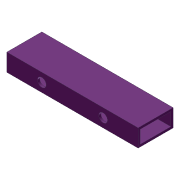
# Autodesk Inventor part: SpatulaPivotMount
Saved by Autodesk Inventor 2012 (Build 160160000, 160)
## iProperties
Created: 2013-01-18
Part Number: SpatulaPivotMount
Material: Aluminum-6061
Document SubType Name: Modeling
Designer: JesseK
Density: 2.71 g/cm^3
Mass: 228.984 g
Surface Area: 541.128 cm^2
Volume: 84.4958 cm^3
Author: JesseK
Autodesk Inventor part; units mm, degrees
ref_plane "YZ Plane" through (0, 0, 0) normal (1, 0, 0) x (0, 1, 0)
ref_plane "XZ Plane" through (0, 0, 0) normal (0, 1, 0) x (-1, 0, 0)
ref_plane "XY Plane" through (0, 0, 0) normal (0, 0, 1) x (1, 0, 0)
sketch "Sketch1" plane through (0, 0, 0) normal (0, 0, 1) x (1, 0, 0)
  line L0 (0, 0) -> (190.5, 0)
  line L1 (190.5, 0) -> (190.5, 25.4)
  line L2 (190.5, 25.4) -> (0, 25.4)
  line L3 (0, 25.4) -> (0, 0)
  dimension "d0" = 190.5
  dimension "d1" = 25.4
  constraints: 8 end point, 2 parallel, 1 horizontal, 1 perpendicular
  measures "d0" distance of L0.start L0.end
  measures "d1" distance of L2.end L0.start
extrude "Extrusion1" add sketch "Sketch1" along normal blind 50.8
shell "Shell1" thickness 3.175 removed faces 2 at (0, 16.9333, 33.8667) at (190.5, 8.4667, 16.9333)
sketch "Sketch4" plane through (0, 0, 0) normal (0, 0, -1) x (-1, 0, 0)
  line L0 (0, 25.4) -> (0, 0) projected
  line L1 (-190.5, 25.4) -> (0, 25.4) projected
  line L2 (-190.5, 0) -> (-190.5, 25.4) projected
  circle A0 centre (-139.7, 12.7) radius 3.175
  circle A1 centre (-50.8, 12.7) radius 3.175
  dimension "d5" = 50.8
  dimension "d6" = 50.8
  dimension "d7" = 12.7
  dimension "d8" = 12.7
  dimension "d9" = 6.35
  constraints: 2 centre point, 1 equal radius
  measures "d5" distance from line of L0 A1.centre
  measures "d6" distance from line of L2 A0.centre
  measures "d7" distance from line of L1 A0.centre
  measures "d8" distance from line of L1 A1.centre
  measures "d9" diameter of A1
extrude "Extrusion2" cut sketch "Sketch4" against normal through all
sketch "Sketch5" plane through (0, 0, 50.8) normal (0, 0, 1) x (1, 0, 0)
  circle A0 centre (50.8, 12.7) radius 3.175 projected
  circle A1 centre (139.7, 12.7) radius 3.175 projected
  circle A2 centre (50.8, 12.7) radius 6.35
  circle A3 centre (139.7, 12.7) radius 6.35
  dimension "d12" = 12.7
  dimension "d13" = 12.7
  constraints: 2 centre point, 2 coincident
  measures "d12" diameter of A3
  measures "d13" diameter of A2
extrude "Extrusion3" cut sketch "Sketch5" against normal up to next
body "Solid1"
